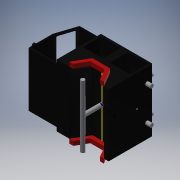
# Autodesk Inventor part: PuertaAtras
Saved by Autodesk Inventor 2017 (Build 210142000, 142)
## iProperties
Part Number: PuertaAtras
Material: Genérico
Document SubType Name: Modeling
Designer: Ghost
Density: 1 g/cm^3
Appearance: Valor por defecto
Author: Ghost
Autodesk Inventor part; units mm, degrees
ref_plane "YZ Plane" through (0, 0, 0) normal (1, 0, 0) x (0, 1, 0)
ref_plane "XZ Plane" through (0, 0, 0) normal (0, 1, 0) x (-1, 0, 0)
sketch "Boceto1" plane through (0, 0, 0) normal (0, 0, 1) x (1, 0, 0)
  line L0 (0, 0) -> (0, 49.6834)
  line L1 (0.0978, 50.3011) -> (13.4493, 91.4177)
  line L2 (15.3516, 92.8) -> (165.8982, 92.8)
  line L3 (167.8982, 90.8) -> (167.8982, 0)
  line L4 (167.8982, 0) -> (0, 0)
  line L5 (58.8982, 92.8) -> (58.8982, 0)
  line L6 (85.3982, 0) -> (102.5709, 29.7439)
  line L7 (104.3029, 30.7439) -> (138.9935, 30.7439)
  line L8 (140.7256, 29.7439) -> (157.8982, 0)
  line L9 (93.3982, 0) -> (106.0709, 21.9497)
  line L10 (107.8029, 22.9497) -> (135.4935, 22.9497)
  line L11 (137.2256, 21.9497) -> (149.8982, 0)
  arc A0 (167.8982, 90.8) -> (165.8982, 92.8) centre (165.8982, 90.8) ccw
  arc A1 (15.3516, 92.8) -> (13.4493, 91.4177) centre (15.3516, 90.8) ccw
  arc A2 (140.7256, 29.7439) -> (138.9935, 30.7439) centre (138.9935, 28.7439) ccw
  arc A3 (104.3029, 30.7439) -> (102.5709, 29.7439) centre (104.3029, 28.7439) ccw
  arc A4 (107.8029, 22.9497) -> (106.0709, 21.9497) centre (107.8029, 20.9497) ccw
  arc A5 (137.2256, 21.9497) -> (135.4935, 22.9497) centre (135.4935, 20.9497) ccw
  arc A6 (0.0978, 50.3011) -> (0, 49.6834) centre (2, 49.6834) ccw
  line L12 (63.8982, 51.9961) -> (63.8982, 85.8)
  line L13 (65.8982, 87.8) -> (103.8982, 87.8)
  line L14 (105.8982, 85.8) -> (105.8982, 51.9961)
  line L15 (103.8982, 49.9961) -> (65.8982, 49.9961)
  line L16 (122.8982, 49.9961) -> (160.8982, 49.9961)
  line L17 (162.8982, 51.9961) -> (162.8982, 85.8)
  line L18 (160.8982, 87.8) -> (122.8982, 87.8)
  line L19 (120.8982, 85.8) -> (120.8982, 51.9961)
  arc A7 (105.8982, 85.8) -> (103.8982, 87.8) centre (103.8982, 85.8) ccw
  arc A8 (65.8982, 87.8) -> (63.8982, 85.8) centre (65.8982, 85.8) ccw
  arc A9 (63.8982, 51.9961) -> (65.8982, 49.9961) centre (65.8982, 51.9961) ccw
  arc A10 (103.8982, 49.9961) -> (105.8982, 51.9961) centre (103.8982, 51.9961) ccw
  arc A11 (120.8982, 51.9961) -> (122.8982, 49.9961) centre (122.8982, 51.9961) ccw
  arc A12 (122.8982, 87.8) -> (120.8982, 85.8) centre (122.8982, 85.8) ccw
  arc A13 (162.8982, 85.8) -> (160.8982, 87.8) centre (160.8982, 85.8) ccw
  arc A14 (160.8982, 49.9961) -> (162.8982, 51.9961) centre (160.8982, 51.9961) ccw
  line L20 (15.3516, 90.8) -> (56.8982, 90.8)
  line L21 (56.8982, 90.8) -> (56.8982, 2)
  line L22 (56.8982, 2) -> (2, 2)
  line L23 (2, 2) -> (2, 49.6834)
  line L24 (2, 49.6834) -> (15.3516, 90.8)
  point P0 (0, 50)
  point P1 (13.8982, 92.8)
  point P2 (167.8982, 92.8)
  point P3 (103.1482, 30.7439)
  point P4 (140.1482, 30.7439)
  point P5 (106.6482, 22.9497)
  point P6 (136.6482, 22.9497)
  point P7 (63.8982, 49.9961)
  point P8 (105.8982, 49.9961)
  point P9 (0.0246, 49.9961)
  point P10 (120.8982, 49.9961)
  dimension "d29" = 154
  dimension "d30" = 92.8
  dimension "d31" = 45
  dimension "d32" = 50
  dimension "d33" = 45
  dimension "d34" = 37
  dimension "d35" = 35.5
  dimension "d37" = 10
  dimension "d38" = 60
  dimension "d39" = 30
  dimension "d40" = 8
  dimension "d41" = 8
  dimension "d42" = 2
  dimension "d43" = 2
  dimension "d44" = 2
  dimension "d51" = 5
  dimension "d52" = 5
  dimension "d53" = 5
  dimension "d54" = 5
  dimension "d55" = 15
  dimension "d56" = 2
  dimension "d57" = 2
  dimension "d58" = 2
  dimension "d59" = 2
  dimension "d60" = 2
  dimension "d61" = 2
  constraints: 50 end point, 31 point on circle, 30 tangent, 26 point on line, 15 centre point, 11 equal radius, 7 parallel, 5 vertical, 4 horizontal, 2 collinear, 2 equal length, 2 horizontal alignment, 2 perpendicular
  measures "d29" distance of point (13.898, 92.8) point (167.898, 92.8)
  measures "d30" distance of point (167.898, 92.8) L3.end
  measures "d31" distance of point (0, 50) point (13.898, 92.8)
  measures "d32" distance of L0.start point (0, 50)
  measures "d33" distance from line of L5 point (13.898, 92.8)
  measures "d34" distance of point (103.148, 30.744) point (140.148, 30.744)
  measures "d35" distance of L6.start point (103.148, 30.744)
  measures "d37" distance of L3.end L8.end
  measures "d38" angle of L4 L6
  measures "d39" distance of point (106.648, 22.95) point (136.648, 22.95)
  measures "d40" distance of L6.start L9.start
  measures "d41" distance of L8.end L11.end
  measures "d42" radius of A0
  measures "d43" radius of A1
  measures "d44" radius of A2
  measures "d51" distance between parallel lines of L2 L13
  measures "d52" distance between parallel lines of L12 L5
  measures "d53" distance between parallel lines of L3 L17
  measures "d54" distance between parallel lines of L2 L18
  measures "d55" distance between parallel lines of L19 L14
  measures "d56" radius of A7
  measures "d57" distance between parallel lines of L2 L20
  measures "d58" distance between parallel lines of L5 L21
  measures "d59" distance between parallel lines of L1 L24
  measures "d60" distance between parallel lines of L0 L23
  measures "d61" distance between parallel lines of L4 L22
extrude "Extrusión7" add sketch "Boceto1" along normal blind 10 contours L5 L2 A0 L3 L4 L8 A2 L7 A3 L6
extrude "Extrusión8" add sketch "Boceto1" along normal blind 2 contours L0 A6 L1 A1 L2 L5 L4
extrude "Extrusión9" add sketch "Boceto1" against normal blind 121.4 contours L5 L2 A0 L3 L4 L8 A2 L7 A3 L6
extrude "Extrusión10" add sketch "Boceto1" against normal blind 113.4 contours L0 A6 L1 A1 L2 L5 L4
sketch "Boceto4" plane through (0, 0, 10) normal (0, 0, 1) x (1, 0, 0)
  line L0 (85.3982, 0) -> (102.5709, 29.7439) projected
  line L1 (104.3029, 30.7439) -> (138.9935, 30.7439) projected
  arc A0 (104.3029, 30.7439) -> (102.5709, 29.7439) centre (104.3029, 28.7439) ccw projected
  arc A1 (122.8982, 87.8) -> (120.8982, 85.8) centre (122.8982, 85.8) ccw projected
  line L2 (122.8982, 87.8) -> (160.8982, 87.8) projected
  arc A2 (162.8982, 85.8) -> (160.8982, 87.8) centre (160.8982, 85.8) ccw projected
  line L3 (162.8982, 85.8) -> (162.8982, 51.9961) projected
  arc A3 (160.8982, 49.9961) -> (162.8982, 51.9961) centre (160.8982, 51.9961) ccw projected
  line L4 (160.8982, 49.9961) -> (122.8982, 49.9961) projected
  arc A4 (120.8982, 51.9961) -> (122.8982, 49.9961) centre (122.8982, 51.9961) ccw projected
  line L5 (120.8982, 51.9961) -> (120.8982, 85.8) projected
  arc A5 (103.8982, 49.9961) -> (105.8982, 51.9961) centre (103.8982, 51.9961) ccw projected
  line L6 (103.8982, 49.9961) -> (65.8982, 49.9961) projected
  arc A6 (63.8982, 51.9961) -> (65.8982, 49.9961) centre (65.8982, 51.9961) ccw projected
  line L7 (63.8982, 51.9961) -> (63.8982, 85.8) projected
  arc A7 (65.8982, 87.8) -> (63.8982, 85.8) centre (65.8982, 85.8) ccw projected
  line L8 (65.8982, 87.8) -> (103.8982, 87.8) projected
  arc A8 (105.8982, 85.8) -> (103.8982, 87.8) centre (103.8982, 85.8) ccw projected
  line L9 (105.8982, 85.8) -> (105.8982, 51.9961) projected
  line L10 (167.8982, 0) -> (167.8982, 90.8) projected
  arc A9 (167.8982, 90.8) -> (165.8982, 92.8) centre (165.8982, 90.8) ccw projected
  line L11 (165.8982, 92.8) -> (58.8982, 92.8) projected
  line L12 (58.8982, 92.8) -> (58.8982, 0) projected
  line L13 (58.8982, 0) -> (85.3982, 0) projected
  line L14 (85.3982, 0) -> (102.5709, 29.7439) projected
  arc A10 (104.3029, 30.7439) -> (102.5709, 29.7439) centre (104.3029, 28.7439) ccw projected
  line L15 (104.3029, 30.7439) -> (138.9935, 30.7439) projected
  arc A11 (140.7256, 29.7439) -> (138.9935, 30.7439) centre (138.9935, 28.7439) ccw projected
  line L16 (140.7256, 29.7439) -> (157.8982, 0) projected
  line L17 (157.8982, 0) -> (167.8982, 0) projected
  line L18 (93.3982, 0) -> (106.0709, 21.9497) projected
  arc A12 (107.8029, 22.9497) -> (106.0709, 21.9497) centre (107.8029, 20.9497) ccw projected
  line L19 (107.8029, 22.9497) -> (135.4935, 22.9497) projected
  arc A13 (137.2256, 21.9497) -> (135.4935, 22.9497) centre (135.4935, 20.9497) ccw projected
  line L20 (137.2256, 21.9497) -> (149.8982, 0) projected
  line L21 (167.8982, 0) -> (0, 0) projected
  constraints: 1 other
extrude "Extrusión11" add sketch "Boceto4" along normal blind 9 contours L0 A0 L1 A11 L16 L21 L20 A13 L19 A12 L18
sketch "Boceto5" plane through (0, 0, -121.4) normal (0, 0, -1) x (-1, 0, 0)
  line L0 (-157.8982, 0) -> (-140.7256, 29.7439) projected
  arc A0 (-138.9935, 30.7439) -> (-140.7256, 29.7439) centre (-138.9935, 28.7439) ccw projected
  line L1 (-138.9935, 30.7439) -> (-104.3029, 30.7439) projected
  arc A1 (-102.5709, 29.7439) -> (-104.3029, 30.7439) centre (-104.3029, 28.7439) ccw projected
  line L2 (-102.5709, 29.7439) -> (-85.3982, 0) projected
  line L3 (-93.3982, 0) -> (-106.0709, 21.9497) projected
  line L4 (-167.8982, 0) -> (0, 0) projected
  line L5 (-107.8029, 22.9497) -> (-135.4935, 22.9497) projected
  arc A2 (-135.4935, 22.9497) -> (-137.2256, 21.9497) centre (-135.4935, 20.9497) ccw projected
  line L6 (-137.2256, 21.9497) -> (-149.8982, 0) projected
  point P0 (-106.6482, 22.9497)
  point P1 (-136.6482, 22.9497)
sketch "Boceto6" plane through (0, 0, -121.4) normal (0, 0, -1) x (-1, 0, 0)
  line L0 (-167.8982, 90.8) -> (-167.8982, 0) projected
  arc A0 (-122.8982, 49.9961) -> (-120.8982, 51.9961) centre (-122.8982, 51.9961) ccw projected
  line L1 (-122.8982, 49.9961) -> (-160.8982, 49.9961) projected
  arc A1 (-162.8982, 51.9961) -> (-160.8982, 49.9961) centre (-160.8982, 51.9961) ccw projected
  line L2 (-162.8982, 51.9961) -> (-162.8982, 85.8) projected
  arc A2 (-160.8982, 87.8) -> (-162.8982, 85.8) centre (-160.8982, 85.8) ccw projected
  line L3 (-160.8982, 87.8) -> (-122.8982, 87.8) projected
  arc A3 (-120.8982, 85.8) -> (-122.8982, 87.8) centre (-122.8982, 85.8) ccw projected
  line L4 (-120.8982, 85.8) -> (-120.8982, 51.9961) projected
  arc A4 (-103.8982, 87.8) -> (-105.8982, 85.8) centre (-103.8982, 85.8) ccw projected
  line L5 (-103.8982, 87.8) -> (-65.8982, 87.8) projected
  arc A5 (-63.8982, 85.8) -> (-65.8982, 87.8) centre (-65.8982, 85.8) ccw projected
  line L6 (-63.8982, 85.8) -> (-63.8982, 51.9961) projected
  arc A6 (-65.8982, 49.9961) -> (-63.8982, 51.9961) centre (-65.8982, 51.9961) ccw projected
  line L7 (-65.8982, 49.9961) -> (-103.8982, 49.9961) projected
  arc A7 (-105.8982, 51.9961) -> (-103.8982, 49.9961) centre (-103.8982, 51.9961) ccw projected
  line L8 (-105.8982, 51.9961) -> (-105.8982, 85.8) projected
  line L9 (-167.8982, 90.8) -> (-167.8982, 0) projected
  line L10 (-167.8982, 0) -> (-157.8982, 0) projected
  line L11 (-157.8982, 0) -> (-140.7256, 29.7439) projected
  arc A8 (-138.9935, 30.7439) -> (-140.7256, 29.7439) centre (-138.9935, 28.7439) ccw projected
  line L12 (-138.9935, 30.7439) -> (-104.3029, 30.7439) projected
  arc A9 (-102.5709, 29.7439) -> (-104.3029, 30.7439) centre (-104.3029, 28.7439) ccw projected
  line L13 (-102.5709, 29.7439) -> (-85.3982, 0) projected
  line L14 (-85.3982, 0) -> (-58.8982, 0) projected
  line L15 (-58.8982, 92.8) -> (-165.8982, 92.8) projected
  arc A10 (-165.8982, 92.8) -> (-167.8982, 90.8) centre (-165.8982, 90.8) ccw projected
  line L16 (-93.3982, 0) -> (-106.0709, 21.9497) projected
  line L17 (-85.3982, 0) -> (-93.3982, 0) projected
  line L18 (-85.3982, 0) -> (-102.5709, 29.7439) projected
  arc A11 (-102.5709, 29.7439) -> (-104.3029, 30.7439) centre (-104.3029, 28.7439) ccw projected
  line L19 (-104.3029, 30.7439) -> (-138.9935, 30.7439) projected
  arc A12 (-138.9935, 30.7439) -> (-140.7256, 29.7439) centre (-138.9935, 28.7439) ccw projected
  line L20 (-140.7256, 29.7439) -> (-157.8982, 0) projected
  line L21 (-149.8982, 0) -> (-157.8982, 0) projected
  line L22 (-137.2256, 21.9497) -> (-149.8982, 0) projected
  arc A13 (-135.4935, 22.9497) -> (-137.2256, 21.9497) centre (-135.4935, 20.9497) ccw projected
  line L23 (-107.8029, 22.9497) -> (-135.4935, 22.9497) projected
  arc A14 (-106.0709, 21.9497) -> (-107.8029, 22.9497) centre (-107.8029, 20.9497) ccw projected
  line L24 (-58.8982, 0) -> (-58.8982, 92.8) projected
  point P0 (0, 0)
extrude "Extrusión12" add sketch "Boceto6" along normal blind 9 contours L11 A8 L12 A9 L13 L17 L16 A14 L23 A13 L22 L21
sketch "Boceto7" plane through (0, 0, 2) normal (-1, 0, 0) x (0, 0, 1)
  circle A0 centre (-105.4, 20) radius 4
  circle A1 centre (-10, 20) radius 4
  line L0 (0, 49.6834) -> (0, 0) projected
  line L1 (0, 0) -> (-115.4, 0) projected
  line L2 (-115.4, 0) -> (-115.4, 49.6834) projected
  point P0 (-2, 0)
  dimension "d80" = 10
  dimension "d81" = 8
  dimension "d82" = 20
  dimension "d83" = 10
  dimension "d135" = 115.4
  constraints: 2 centre point, 1 equal radius, 1 horizontal alignment
  measures "d80" distance from line of L0 A1.centre
  measures "d81" diameter of A1
  measures "d82" distance from line of L1 A1.centre
  measures "d83" distance from line of L2 A0.centre
  measures "d135" distance of L0.end L1.end
extrude "Extrusión13" add sketch "Boceto7" along normal blind 10
sketch "Boceto8" plane through (0.0978, 50.3011, -113.4) normal (-0.9511111, 0.3088489, 0) x (0, 0, 1)
  line L0 (7.05, 5) -> (108.35, 5)
  line L1 (110.4, 7.05) -> (110.4, 36.1801)
  line L2 (108.35, 38.2301) -> (7.05, 38.2301)
  line L3 (5, 36.1801) -> (5, 7.05)
  line L4 (0, -28.397) -> (0, 56.0617) projected
  line L5 (0, -0.6177) -> (115.4, -0.6177) projected
  line L6 (115.4, 43.2301) -> (115.4, 0) projected
  line L7 (0, 43.2301) -> (115.4, 43.2301) projected
  arc A0 (7.05, 38.2301) -> (5, 36.1801) centre (7.05, 36.1801) ccw
  arc A1 (110.4, 36.1801) -> (108.35, 38.2301) centre (108.35, 36.1801) ccw
  arc A2 (108.35, 5) -> (110.4, 7.05) centre (108.35, 7.05) ccw
  arc A3 (5, 7.05) -> (7.05, 5) centre (7.05, 7.05) ccw
  line L8 (0, 0) -> (115.4, 0) projected
  point P0 (113.4, -47.8721)
  dimension "d92" = 2.05
  dimension "d93" = 5
  dimension "d94" = 5
  dimension "d95" = 5
  dimension "d96" = 5
  dimension "d136" = 33.2301
  dimension "d137" = 105.4
  constraints: 8 end point, 8 point on circle, 8 tangent, 4 centre point, 3 equal radius, 2 parallel, 1 horizontal, 1 vertical
  measures "d92" radius of A0
  measures "d93" distance between parallel lines of L3 L4
  measures "d94" distance between parallel lines of L7 L2
  measures "d95" distance between parallel lines of L6 L1
  measures "d96" distance between parallel lines of L8 L0
  measures "d136" distance between parallel lines of L0 L2
  measures "d137" distance between parallel lines of L1 L3
extrude "Extrusión15" cut sketch "Boceto8" against normal blind 2 contours A3 L3 A0 L2 A1 L1 A2 L0
sketch "Boceto9" plane through (58.8982, 0, 10) normal (-1, 0, 0) x (0, 0, 1)
  circle A0 centre (-4, 89.8) radius 1.5
  circle A1 centre (-4, 10) radius 1.5
  line L0 (-8, 92.8) -> (0, 92.8) projected
  line L1 (-8, 91.4177) -> (-8, 50.3011) projected
  line L2 (-8, 0) -> (0, 0) projected
  point P0 (-10, 0)
  dimension "d99" = 3
  dimension "d100" = 3
  dimension "d101" = 4
  dimension "d102" = 10
  constraints: 2 centre point, 1 equal radius, 1 vertical alignment
  measures "d99" diameter of A0
  measures "d100" distance from line of L0 A0.centre
  measures "d101" distance from line of L1 A0.centre
  measures "d102" distance from line of L2 A1.centre
extrude "Extrusión16" cut sketch "Boceto9" against normal blind 10
sketch "Boceto10" plane through (58.8982, 0, -121.4) normal (-1, 0, 0) x (0, 0, 1)
  circle A0 centre (4, 89.8) radius 1.5
  circle A1 centre (4, 10) radius 1.5
  line L0 (8, 92.8) -> (0, 92.8) projected
  line L1 (8, 50.3011) -> (8, 91.4177) projected
  line L2 (8, 0) -> (0, 0) projected
  point P0 (121.4, 0)
  dimension "d105" = 3
  dimension "d106" = 4
  dimension "d107" = 10
  dimension "d108" = 3
  constraints: 2 centre point, 1 equal radius, 1 vertical alignment
  measures "d105" distance from line of L0 A0.centre
  measures "d106" distance from line of L1 A0.centre
  measures "d107" distance from line of L2 A1.centre
  measures "d108" diameter of A0
extrude "Extrusión17" cut sketch "Boceto10" against normal blind 10
sketch "Boceto11" plane through (104.3029, 30.7439, 10) normal (0, -1, 0) x (1, 0, 0)
  line L0 (18.5953, -131.4) -> (18.5953, 0) projected
  circle A0 centre (18.5953, -65.7) radius 4
  point P0 (-104.3029, -10)
  dimension "d111" = 8
  constraints: 1 centre point, 1 midpoint
  measures "d111" diameter of A0
extrude "Extrusión18" add sketch "Boceto11" along normal blind 40
ref_plane "Plano de trabajo1" through (0, 0, -55.7) normal (0, 0, 1) x (1, 0, 0)
sketch "Boceto13" plane through (0, 0, -55.7) normal (0, 0, 1) x (1, 0, 0)
  line L0 (118.8982, -9.2561) -> (126.8982, -9.2561) projected
  circle A0 centre (122.8982, -9.2561) radius 4
  point P0 (0, 0)
  dimension "d115" = 8
  constraints: 1 centre point, 1 midpoint
  measures "d115" diameter of A0
extrude "Extrusión19" add sketch "Boceto13" along normal mid plane 131.4
sketch "Boceto14" plane through (58.8982, 92.8, 10) normal (0, 1, 0) x (1, 0, 0)
  circle A0 centre (97, 30) radius 4
  circle A1 centre (97, 101.4) radius 4
  line L0 (107, 0) -> (0, 0) projected
  line L1 (0, 131.4) -> (107, 131.4) projected
  line L2 (107, 131.4) -> (107, 0) projected
  point P0 (-58.8982, 10)
  dimension "d118" = 8
  dimension "d119" = 30
  dimension "d120" = 30
  dimension "d121" = 10
  constraints: 2 centre point, 1 equal radius, 1 vertical alignment
  measures "d118" diameter of A0
  measures "d119" distance from line of A0.centre L0
  measures "d120" distance from line of L1 A1.centre
  measures "d121" distance from line of L2 A0.centre
extrude "Extrusión20" add sketch "Boceto14" along normal blind 10
sketch "Boceto15" plane through (167.8982, 0, 10) normal (1, 0, 0) x (0, 0, -1)
  circle A0 centre (30, 80.8) radius 4
  circle A1 centre (101.4, 80.8) radius 4
  line L0 (0, 0) -> (0, 90.8) projected
  line L1 (131.4, 90.8) -> (131.4, 0) projected
  line L2 (131.4, 90.8) -> (0, 90.8) projected
  point P0 (10, 0)
  dimension "d124" = 30
  dimension "d125" = 30
  dimension "d126" = 8
  dimension "d127" = 10
  constraints: 2 centre point, 1 equal radius, 1 horizontal alignment
  measures "d124" distance from line of L0 A0.centre
  measures "d125" distance from line of L1 A1.centre
  measures "d126" diameter of A0
  measures "d127" distance from line of L2 A0.centre
extrude "Extrusión21" add sketch "Boceto15" along normal blind 10
sketch "Boceto16" plane through (167.8982, 0, 10) normal (1, 0, 0) x (0, 0, -1)
  circle A0 centre (65.7, 60) radius 1.5
  line L0 (131.4, 90.8) -> (131.4, 0) projected
  line L1 (0, 0) -> (131.4, 0) projected
  point P0 (10, 0)
  dimension "d130" = 3
  dimension "d131" = 65.7
  dimension "d132" = 60
  constraints: 1 centre point
  measures "d130" diameter of A0
  measures "d131" distance from line of L0 A0.centre
  measures "d132" distance from line of L1 A0.centre
extrude "Extrusión22" cut sketch "Boceto16" against normal blind 10
